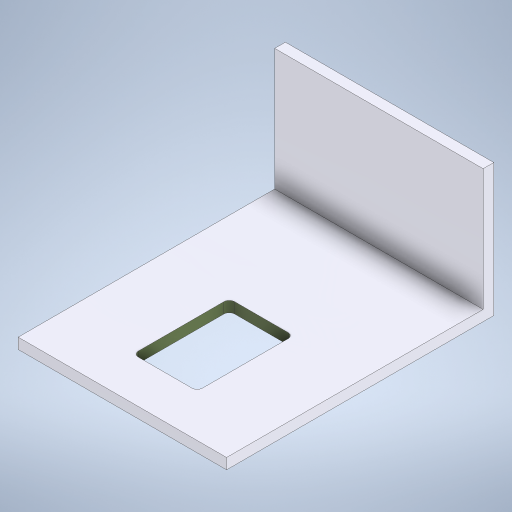
# Autodesk Inventor part: Kamera 2
Saved by Autodesk Inventor 2023 (Build 270158000, 158)
## iProperties
Created: 2025-05-30
Part Number: Kamera 2
Material: Generic
Document SubType Name: Modeling
Designer: ASUS
Density: 1 g/cm^3
Appearance: Default
Author: ASUS
Autodesk Inventor part; units mm, degrees
ref_plane "YZ Plane" through (0, 0, 0) normal (1, 0, 0) x (0, 1, 0)
ref_plane "XZ Plane" through (0, 0, 0) normal (0, 1, 0) x (-1, 0, 0)
ref_plane "XY Plane" through (0, 0, 0) normal (0, 0, 1) x (1, 0, 0)
sketch "Sketch1" plane through (0, 0, 0) normal (0, 0, 1) x (1, 0, 0)
  line L0 (0, 0) -> (39, 0)
  line L1 (39, 0) -> (39, 24.8)
  line L2 (39, 24.8) -> (0, 24.8)
  line L3 (0, 24.8) -> (0, 0)
  dimension "d0" = 39
  dimension "d1" = 24.8
  constraints: 8 end point, 2 parallel, 1 horizontal, 1 perpendicular
  measures "d0" distance of L2.end L1.end
  measures "d1" distance of L1.end L0.end
extrude "Extrusion1" add sketch "Sketch1" along normal blind 2
sketch "Sketch2" plane through (0, 0, 2) normal (0, 0, 1) x (1, 0, 0)
  line L0 (0, 24.8) -> (0, 0) projected
  line L1 (0, 0) -> (39, 0)
  line L2 (39, 0) -> (39, 2)
  line L3 (39, 2) -> (0, 2)
  line L4 (0, 2) -> (0, 0)
  dimension "d4" = 39
  dimension "d5" = 2
  constraints: 8 end point, 2 parallel, 1 horizontal, 1 perpendicular
  measures "d4" distance of L3.end L2.end
  measures "d5" distance of L2.end L1.end
extrude "Extrusion2" add sketch "Sketch2" along normal blind 48
sketch "Sketch3" plane through (0, 0, 0) normal (0, -1, 0) x (1, 0, 0)
  line L0 (0, 0) -> (39, 0) projected
  line L1 (19.5, 24) -> (24.5, 24)
  line L2 (25.5, 25) -> (25.5, 41)
  line L3 (24.5, 42) -> (14.5, 42)
  line L4 (13.5, 41) -> (13.5, 25)
  line L5 (14.5, 24) -> (19.5, 24)
  arc A0 (14.5, 42) -> (13.5, 41) centre (14.5, 41) ccw
  arc A1 (24.5, 24) -> (25.5, 25) centre (24.5, 25) ccw
  arc A2 (25.5, 41) -> (24.5, 42) centre (24.5, 41) ccw
  arc A3 (13.5, 25) -> (14.5, 24) centre (14.5, 25) ccw
  point P0 (25.5, 24)
  point P1 (25.5, 42)
  point P2 (13.5, 42)
  point P3 (13.5, 24)
  dimension "d9" = 6
  dimension "d10" = 18
  dimension "d11" = 12
  dimension "d12" = 18
  dimension "d13" = 1
  constraints: 10 end point, 8 point on circle, 8 point on line, 8 tangent, 4 centre point, 3 equal radius, 2 perpendicular, 1 horizontal, 1 vertical
  measures "d9" distance of L1.start point (25.5, 24)
  measures "d10" distance of point (25.5, 24) point (25.5, 42)
  measures "d11" distance of point (25.5, 42) point (13.5, 42)
  measures "d12" distance of point (13.5, 42) point (13.5, 24)
  measures "d13" radius of A0
extrude "Extrusion3" cut sketch "Sketch3" against normal blind 48
body "Solid1"
